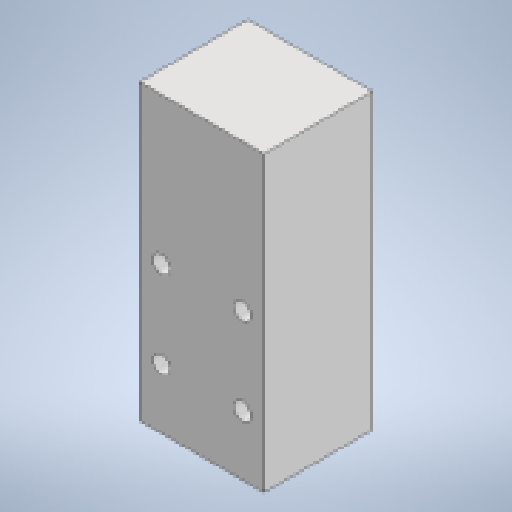
# Autodesk Inventor part: основа_каретки
Saved by Autodesk Inventor 2023.1 (Build 271208000, 208)
## iProperties
Created: 2026-01-04
Part Number: основа_каретки
Material: Типовые
Document SubType Name: Modeling
Designer: DELL
Density: 1 g/cm^3
Appearance: По умолчанию
Author: DELL
Autodesk Inventor part; units mm, degrees
ref_plane "YZ Plane" through (0, 0, 0) normal (1, 0, 0) x (0, 1, 0)
ref_plane "XZ Plane" through (0, 0, 0) normal (0, 1, 0) x (-1, 0, 0)
ref_plane "XY Plane" through (0, 0, 0) normal (0, 0, 1) x (1, 0, 0)
sketch "Эскиз1" plane through (0, 0, 0) normal (0, 0, 1) x (1, 0, 0)
  circle A0 centre (7.5, -22.95) radius 1.5 construction
  circle A1 centre (-7.5, -22.95) radius 1.5 construction
  circle A2 centre (-7.5, -6.95) radius 1.5 construction
  circle A3 centre (7.5, -6.95) radius 1.5 construction
  line L0 (-7.5, -6.95) -> (7.5, -22.95) construction
  line L1 (-11.5, -34) -> (11.5, -34)
  line L2 (11.5, -34) -> (11.5, 4.1)
  line L3 (11.5, 4.1) -> (-11.5, 4.1)
  line L4 (-11.5, 4.1) -> (-11.5, -34)
  line L5 (0, 4.1) -> (0, -34) construction
  line L6 (-7.5, -6.95) -> (7.5, -6.95) construction
  line L7 (0, -6.95) -> (0, -14.7883) construction
  line L8 (9, -34) -> (-9, -34) construction
  circle A4 centre (7.5, -6.95) radius 1.6
  circle A5 centre (-7.5, -22.95) radius 1.6
  circle A6 centre (7.5, -22.95) radius 1.6
  circle A7 centre (-7.5, -6.95) radius 1.6
  line L9 (9, 4.1) -> (-9, 4.1) construction
  point P0 (0, 0)
  point P1 (0, -10.8692)
  point P2 (0, -34)
  point P3 (0, 4.1)
  dimension "d0" = 4
  dimension "d2" = 3.2
  dimension "d3" = 3.2
  dimension "d4" = 3.2
  dimension "d5" = 3.2
  constraints: 16 end point, 8 midpoint, 4 centre point, 4 coincident, 2 horizontal, 2 parallel, 1 collinear, 1 perpendicular, 1 point on line
  measures "d0" distance from line of L6.end L2
  measures "d2" diameter of A4
  measures "d3" diameter of A5
  measures "d4" diameter of A6
  measures "d5" diameter of A7
extrude "Выдавливание1" add sketch "Эскиз1" along normal blind 20
